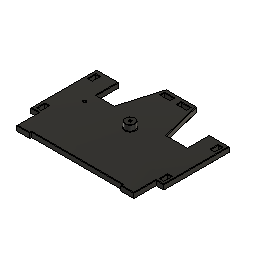
Rama stanga (Autodesk Fusion 360 design; units mm, degrees)
part number: 2026-05-28-04-13-53-551
Autodesk Fusion 360 part; units mm, degrees
sketch "Sketch1" plane through (0, 0, 0) normal (0, 0, 1) x (1, 0, 0)
  line L0 (27.8497, 75.8381) -> (51.8497, 75.8381)
  line L1 (51.8497, 75.8381) -> (51.8497, 51.1381)
  line L2 (51.8497, 51.1381) -> (71.8497, 51.1381)
  line L3 (71.8497, 51.1381) -> (84.8497, 95.4381)
  line L4 (84.8497, 95.4381) -> (117.8497, 95.4381)
  line L5 (117.8497, 95.4381) -> (128.8497, 51.4381)
  line L6 (128.8497, 51.4381) -> (151.8497, 51.4381)
  line L7 (151.8497, 51.4381) -> (151.8497, 75.4381)
  line L8 (151.8497, 75.4381) -> (173.8497, 75.4381)
  line L9 (173.8497, 75.4381) -> (173.8497, 3.4381)
  line L10 (173.8497, 3.4381) -> (165.4497, 3.4381)
  line L11 (165.4497, 3.4381) -> (165.4497, -21.0619)
  line L12 (165.4497, -21.0619) -> (151.0497, -21.0619)
  line L13 (151.0497, -21.0619) -> (151.0497, -19.0619)
  line L14 (151.0497, -19.0619) -> (51.0497, -19.0619)
  line L15 (51.0497, -19.0619) -> (51.0497, -21.0619)
  line L16 (51.0497, -21.0619) -> (36.7497, -21.0619)
  line L17 (36.7497, -21.0619) -> (36.7497, 3.4381)
  line L18 (36.7497, 3.4381) -> (27.7497, 3.4381)
  line L19 (27.7497, 3.4381) -> (27.8497, 75.8381)
  line L20 (31.5497, 71.033) -> (35.8497, 71.033)
  line L21 (35.8497, 71.033) -> (35.8497, 62.733)
  line L22 (35.8497, 62.733) -> (31.5497, 62.733)
  line L23 (31.5497, 62.733) -> (31.5497, 71.033)
  line L24 (31.4497, 6.933) -> (35.7497, 6.933)
  line L25 (35.7497, 6.933) -> (35.7497, 15.233)
  line L26 (35.7497, 15.233) -> (31.4497, 15.233)
  line L27 (31.4497, 15.233) -> (31.4497, 6.933)
  line L28 (170.5497, 70.9381) -> (166.2497, 70.9381)
  line L29 (166.2497, 70.9381) -> (166.2497, 62.6381)
  line L30 (166.2497, 62.6381) -> (170.5497, 62.6381)
  line L31 (170.5497, 62.6381) -> (170.5497, 70.9381)
  line L32 (170.5497, 6.9381) -> (166.2497, 6.9381)
  line L33 (166.2497, 6.9381) -> (166.2497, 15.2381)
  line L34 (166.2497, 15.2381) -> (170.5497, 15.2381)
  line L35 (170.5497, 15.2381) -> (170.5497, 6.9381)
  line L36 (86.7497, 91.2381) -> (97.0497, 91.2381)
  line L37 (97.0497, 91.2381) -> (97.0497, 86.9381)
  line L38 (97.0497, 86.9381) -> (86.7497, 86.9381)
  line L39 (86.7497, 86.9381) -> (86.7497, 91.2381)
  line L40 (105.0497, 91.2381) -> (115.3497, 91.2381)
  line L41 (115.3497, 91.2381) -> (115.3497, 86.9381)
  line L42 (115.3497, 86.9381) -> (105.0497, 86.9381)
  line L43 (105.0497, 86.9381) -> (105.0497, 91.2381)
  line L44 (84.8497, 95.4381) -> (101.3497, 95.4381)
  circle A0 centre (101.3497, 38.9381) radius 1.25
  circle A1 centre (101.3497, 38.9381) radius 5.5
  circle A2 centre (51.3497, 38.9381) radius 1.25
  dimension "d1" = 24
  dimension "d2" = 24.7
  dimension "d3" = 20
  dimension "d6" = 33
  dimension "d9" = 23
  dimension "d10" = 24
  dimension "d11" = 22
  dimension "d12" = 72
  dimension "d13" = 8.4
  dimension "d14" = 24.5
  dimension "d15" = 14.4
  dimension "d16" = 2
  dimension "d17" = 100
  dimension "d18" = 2
  dimension "d19" = 14.3
  dimension "d20" = 24.5
  dimension "d21" = 9
  dimension "d24" = 4.3
  dimension "d25" = 8.3
  dimension "d28" = 4.3
  dimension "d29" = 8.3
  dimension "d32" = 4.3
  dimension "d33" = 8.3
  dimension "d36" = 4.3
  dimension "d37" = 8.3
  dimension "d40" = 10.3
  dimension "d41" = 4.3
  dimension "d42" = 8
  dimension "d43" = 10.3
  dimension "d44" = 4.3
  dimension "d45" = 56.5
  dimension "d46" = 2.5
  dimension "d47" = 11
  dimension "d48" = 50
  dimension "d49" = 2.5
  constraint horizontal L0
  constraint perpendicular L0 L1
  constraint perpendicular L1 L2
  constraint perpendicular L6 L7
  constraint perpendicular L7 L8
  constraint perpendicular L8 L9
  constraint perpendicular L9 L10
  constraint perpendicular L10 L11
  constraint perpendicular L11 L12
  constraint vertical L13
  constraint perpendicular L13 L14
  constraint perpendicular L14 L15
  constraint perpendicular L15 L16
  constraint perpendicular L16 L17
  constraint perpendicular L17 L18
  constraint horizontal L20
  constraint vertical L21
  constraint horizontal L22
  constraint vertical L23
  constraint horizontal L24
  constraint vertical L25
  constraint horizontal L26
  constraint vertical L27
  constraint horizontal L28
  constraint vertical L29
  constraint horizontal L30
  constraint vertical L31
  constraint horizontal L32
  constraint vertical L33
  constraint horizontal L34
  constraint vertical L35
  constraint horizontal L36
  constraint vertical L37
  constraint horizontal L38
  constraint vertical L39
  constraint horizontal L40
  constraint vertical L41
  constraint horizontal L42
  constraint vertical L43
  constraint midpoint L4 L44.end
  constraint concentric A0 A1
  measures "d1" distance of L0.start L0.end
  measures "d2" distance of L0.end L1.end
  measures "d3" distance of L1.end L2.end
  measures "d6" distance of L3.end L4.end
  measures "d9" distance of L5.end L6.end
  measures "d10" distance of L6.end L7.end
  measures "d11" distance of L7.end L8.end
  measures "d12" distance of L8.end L9.end
  measures "d13" distance of L9.end L10.end
  measures "d14" distance of L10.end L11.end
  measures "d15" distance of L11.end L12.end
  measures "d16" distance of L12.end L13.end
  measures "d17" distance of L13.end L14.end
  measures "d18" distance of L14.end L15.end
  measures "d19" distance of L15.end L16.end
  measures "d20" distance of L16.end L17.end
  measures "d21" distance of L17.end L18.end
  measures "d24" distance of L20.start L20.end
  measures "d25" distance of L20.start L22.end
  measures "d28" distance of L24.start L24.end
  measures "d29" distance of L24.start L26.end
  measures "d32" distance of L28.start L28.end
  measures "d33" distance of L28.start L30.end
  measures "d36" distance of L32.start L32.end
  measures "d37" distance of L32.start L34.end
  measures "d40" distance of L36.start L36.end
  measures "d41" distance of L36.start L38.end
  measures "d42" distance of L36.end L40.start
  measures "d43" distance of L40.start L40.end
  measures "d44" distance of L40.start L42.end
  measures "d45" distance of L44.end A0.centre
  measures "d46" diameter of A0
  measures "d47" diameter of A1
  measures "d48" distance of A0.centre A2.centre
  measures "d49" diameter of A2
extrude "Extrude1" add sketch "Sketch1" along normal blind 6 contours L0 L1 L2 L3 L4 L5 L6 L7 L8 L9 L10 L11 L12 L13 L14 L15 L16 L17 L18 L19 L44
extrude "Extrude2" add sketch "Sketch1" along normal blind 12.5 contours A1
chamfer "Chamfer1" distance 0.5 angle 45 1 faces at (101.0127, -1.5568, 6)
chamfer "Chamfer2" distance 0.3 angle 45 1 faces at (105.4126, 38.6648, 12.5)
chamfer "Chamfer3" distance 0.5 angle 45 1 faces at (101.0904, -0.141, 0)
